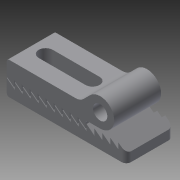
# Autodesk Inventor part: CableClpam
Saved by Autodesk Inventor 2015 (Build 190159000, 159)
## iProperties
Created: 2014-11-13
Part Number: CableClpam
Material: Generic
Document SubType Name: Modeling
Designer: rawrdong
Density: 1 g/cm^3
Appearance: Default
Author: rawrdong
Autodesk Inventor part; units mm, degrees
ref_plane "YZ Plane" through (0, 0, 0) normal (1, 0, 0) x (0, 1, 0)
ref_plane "XZ Plane" through (0, 0, 0) normal (0, 1, 0) x (-1, 0, 0)
ref_plane "XY Plane" through (0, 0, 0) normal (0, 0, 1) x (1, 0, 0)
sketch "Sketch1" plane through (0, 0, 0) normal (0, 1, 0) x (-1, 0, 0)
  line L0 (1.1699, 0) -> (26.6699, 0)
  line L1 (26.6699, 0) -> (26.6699, 2)
  line L2 (26.6699, 2) -> (9.6699, 2)
  line L3 (26.6699, 2) -> (26.6699, 3.3)
  line L4 (26.6699, 3.3) -> (24.9699, 2)
  line L5 (26.6699, 2) -> (24.9699, 2)
  line L6 (24.9699, 2) -> (24.9699, 3.3)
  line L7 (24.9699, 3.3) -> (23.2699, 2)
  line L8 (24.9699, 2) -> (23.2699, 2)
  line L9 (23.2699, 2) -> (23.2699, 3.3)
  line L10 (23.2699, 3.3) -> (21.5699, 2)
  line L11 (23.2699, 2) -> (21.5699, 2)
  line L12 (21.5699, 2) -> (21.5699, 3.3)
  line L13 (21.5699, 3.3) -> (19.8699, 2)
  line L14 (21.5699, 2) -> (19.8699, 2)
  line L15 (19.8699, 2) -> (19.8699, 3.3)
  line L16 (19.8699, 3.3) -> (18.1699, 2)
  line L17 (19.8699, 2) -> (18.1699, 2)
  line L18 (18.1699, 2) -> (18.1699, 3.3)
  line L19 (18.1699, 3.3) -> (16.4699, 2)
  line L20 (18.1699, 2) -> (16.4699, 2)
  line L21 (16.4699, 2) -> (16.4699, 3.3)
  line L22 (16.4699, 3.3) -> (14.7699, 2)
  line L23 (16.4699, 2) -> (14.7699, 2)
  line L24 (14.7699, 2) -> (14.7699, 3.3)
  line L25 (14.7699, 3.3) -> (13.0699, 2)
  line L26 (14.7699, 2) -> (13.0699, 2)
  line L27 (13.0699, 2) -> (13.0699, 3.3)
  line L28 (13.0699, 3.3) -> (11.3699, 2)
  line L29 (13.0699, 2) -> (11.3699, 2)
  line L30 (11.3699, 2) -> (11.3699, 3.3)
  line L31 (11.3699, 3.3) -> (9.6699, 2)
  line L32 (11.3699, 2) -> (9.6699, 2)
  line L33 (9.6699, 2) -> (9.6699, 3.3)
  line L34 (9.6699, 3.3) -> (7.9699, 2)
  line L35 (9.6699, 2) -> (7.9699, 2)
  line L36 (7.9699, 2) -> (7.9699, 3.3)
  line L37 (7.9699, 3.3) -> (6.2699, 2)
  line L38 (7.9699, 2) -> (6.2699, 2)
  line L39 (6.2699, 2) -> (6.2699, 3.3)
  line L40 (6.2699, 3.3) -> (4.5699, 2)
  line L41 (6.2699, 2) -> (4.5699, 2)
  line L42 (4.5699, 2) -> (4.5699, 3.3)
  line L43 (4.5699, 3.3) -> (2.8699, 2)
  line L44 (4.5699, 2) -> (2.8699, 2)
  line L45 (2.8699, 2) -> (2.8699, 3.3)
  line L46 (2.8699, 3.3) -> (1.1699, 2)
  line L47 (2.8699, 2) -> (1.1699, 2)
  line L48 (1.1699, 2) -> (1.1699, 0)
  line L49 (1.1699, 2) -> (26.6699, 2)
  line L50 (26.6699, 2) -> (26.6699, 0)
  line L51 (26.6699, 0) -> (1.1699, 0)
  line L52 (1.1699, 0) -> (1.1699, 2)
  point P0 (0, 0)
  dimension "d7" = 1.3
  dimension "d8" = 2
  dimension "d11" = 1.7
  dimension "d14" = 1.7
  constraints: 106 end point, 3 horizontal, 3 parallel, 3 perpendicular, 1 coincident, 1 collinear, 1 point on line, 1 vertical, 85 other
  measures "d7" distance of L1.end L3.end
  measures "d8" distance of L0.end L1.end
  measures "d11" distance from line of L3 L4.end
  measures "d14" distance of L3.end L7.start
extrude "Extrusion1" add sketch "Sketch1" along normal blind 10
sketch "Sketch2" plane through (0, 10, 0) normal (0, 1, 0) x (1, 0, 0)
  line L0 (-19.8699, -3.3) -> (-18.1699, -2) projected
  line L1 (-18.1699, -2) -> (-18.1699, -3.3) projected
  line L2 (-18.1699, -3.3) -> (-16.4699, -2) projected
  line L3 (-16.4699, -2) -> (-16.4699, -3.3) projected
  line L4 (-16.4699, -3.3) -> (-14.7699, -2) projected
  line L5 (-14.7699, -2) -> (-14.7699, -3.3) projected
  line L6 (-14.7699, -3.3) -> (-13.0699, -2) projected
  line L7 (-13.0699, -2) -> (-13.0699, -3.3) projected
  line L8 (-13.0699, -3.3) -> (-11.3699, -2) projected
  line L9 (-11.3699, -2) -> (-11.3699, -3.3) projected
  line L10 (-11.3699, -3.3) -> (-9.6699, -2) projected
  line L11 (-9.8699, -2.4047) -> (-11.5699, -3.7047)
  line L12 (-11.5699, -3.7047) -> (-11.5699, -2.4047)
  line L13 (-11.5699, -2.4047) -> (-13.2699, -3.7047)
  line L14 (-13.2699, -3.7047) -> (-13.2699, -2.4047)
  line L15 (-13.2699, -2.4047) -> (-14.9699, -3.7047)
  line L16 (-14.9699, -3.7047) -> (-14.9699, -2.4047)
  line L17 (-14.9699, -2.4047) -> (-16.6699, -3.7047)
  line L18 (-16.6699, -3.7047) -> (-16.6699, -2.4047)
  line L19 (-16.6699, -2.4047) -> (-18.3699, -3.7047)
  line L20 (-18.3699, -3.7047) -> (-18.3699, -2.4047)
  line L21 (-18.3699, -2.4047) -> (-20.0699, -3.7047)
  line L22 (-10.9918, -6.9047) -> (-26.6699, -6.9047)
  line L23 (-21.5699, -3.3) -> (-19.8699, -2) projected
  line L24 (-19.8699, -2) -> (-19.8699, -3.3) projected
  line L25 (-20.0699, -2.4047) -> (-20.0699, -3.7047)
  line L26 (-20.0699, -2.4047) -> (-21.7699, -3.7047)
  circle A0 centre (-6.7492, -6.9047) radius 1.525
  circle A1 centre (-6.7492, -6.9047) radius 3
  line L27 (-8.8705, -9.026) -> (-10.9918, -6.9047)
  line L28 (-6.7492, -3.9047) -> (-9.8699, -3.9047)
  line L29 (-9.8699, -2.4047) -> (-9.8699, -3.9047)
  line L30 (-9.6699, -2) -> (-9.6699, -3.3) projected
  line L31 (-26.6699, -3.3) -> (-24.9699, -2) projected
  line L32 (-24.9699, -2) -> (-24.9699, -3.3) projected
  line L33 (-24.9699, -3.3) -> (-23.2699, -2) projected
  line L34 (-23.2699, -2) -> (-23.2699, -3.3) projected
  line L35 (-23.2699, -3.3) -> (-21.5699, -2) projected
  line L36 (-4.5699, -2) -> (-4.5699, -3.3) projected
  line L37 (-21.7699, -2.4047) -> (-23.4699, -3.7047)
  line L38 (-23.4699, -3.7047) -> (-23.4699, -2.4047)
  line L39 (-23.4699, -2.4047) -> (-25.1699, -3.7047)
  line L40 (-25.1699, -3.7047) -> (-25.1699, -2.4047)
  line L41 (-25.1699, -2.4047) -> (-26.6699, -3.5518)
  line L42 (-21.7699, -2.4047) -> (-21.7699, -3.7047)
  line L43 (-6.2699, -2) -> (-6.2699, -3.3) projected
  line L44 (-26.6699, -3.5518) -> (-26.6699, -6.9047)
  dimension "d22" = 0.2
  dimension "d23" = 0.2
  dimension "d53" = 3.05
  dimension "d54" = 6
  dimension "d55" = 0.2
  dimension "d71" = 0.2
  dimension "d76" = 135
  constraints: 48 end point, 7 parallel, 5 horizontal alignment, 2 centre point, 2 horizontal, 2 point on circle, 2 tangent, 1 coincident, 12 other
  measures "d22" distance between parallel lines of L4 L17
  measures "d23" distance between parallel lines of L10 L11
  measures "d53" diameter of A0
  measures "d54" diameter of A1
  measures "d55" distance from line of L11.end L28
  measures "d71" distance between parallel lines of L30 L29
  measures "d76" angle of L22 L27
extrude "Extrusion2" add sketch "Sketch2" against normal blind 10
sketch "Sketch13" plane through (-1.1699, 0, 0) normal (0, 0, -1) x (-1, 0, 0)
  line L0 (25.5, 0) -> (25.5, 10) projected
  line L1 (0, 10) -> (25.5, 10) projected
  circle A0 centre (12.75, 5) radius 1.5
  point P0 (-1.1699, 0)
  point P1 (12.75, 10)
  point P2 (25.5, 5)
  dimension "d73" = 3
  constraints: 2 midpoint, 1 centre point, 1 horizontal alignment, 1 vertical alignment
  measures "d73" diameter of A0
extrude "Extrusion13" cut sketch "Sketch13" against normal up to next
sketch "Sketch4" plane through (-10.302, 0, 6.9047) normal (0, 0, 1) x (1, 0, 0)
  line L0 (-16.3678, 10) -> (-0.6898, 10) projected
  line L1 (-13.0678, 5) -> (-3.0678, 5) construction
  line L2 (-13.0678, 3.5) -> (-3.0678, 3.5)
  line L3 (-3.0678, 6.5) -> (-13.0678, 6.5)
  arc A0 (-13.0678, 6.5) -> (-13.0678, 3.5) centre (-13.0678, 5) ccw
  arc A1 (-3.0678, 3.5) -> (-3.0678, 6.5) centre (-3.0678, 5) ccw
  line L4 (-16.3678, 10) -> (-16.3678, 0) projected
  circle A2 centre (-3.6178, 5) radius 1.5 projected
  point P0 (-8.0678, 5)
  point P1 (-8.0678, 10)
  point P2 (-16.3678, 5)
  dimension "d32" = 3
  dimension "d35" = 10
  constraints: 8 end point, 4 point on circle, 4 tangent, 2 centre point, 2 midpoint, 2 parallel, 1 horizontal alignment, 1 vertical alignment
  measures "d32" distance between parallel lines of L2 L3
  measures "d35" distance of L1.start L1.end
extrude "Extrusion4" cut sketch "Sketch4" against normal up to next
fillet "Fillet5" radius 2.5 1 edges at (-10.9918, 5, 6.9047)
fillet "Fillet6" radius 0.5 3 edges at (-26.6699, 5, 6.9047) (-26.6699, 5, 0) (-9.8699, 5, 3.9047)
fillet "Fillet9" radius 1 2 edges at (-1.1699, 10, 1) (-1.1699, 0, 1)
sketch "Sketch11" plane through (-23.3699, 5.4, 6.5462) normal (0, -1, 0) x (1, 0, 0)
  line L0 (8.4, -2.8415) -> (10, -4.065) projected
  line L1 (8.4, -4.1415) -> (8.4, -2.8415) projected
  line L2 (6.7, -2.8415) -> (8.4, -4.1415) projected
  line L3 (6.7, -4.1415) -> (6.7, -2.8415) projected
  line L4 (5, -2.8415) -> (6.7, -4.1415) projected
  line L5 (5, -4.1415) -> (5, -2.8415) projected
  line L6 (3.3, -2.8415) -> (5, -4.1415) projected
  line L7 (0, 0) -> (0, -2.9179) projected
  line L8 (10, 0) -> (0, 0) projected
  line L9 (10, 0) -> (10, -4.065) projected
  line L10 (3.3, -4.1415) -> (3.3, -2.8415) projected
  line L11 (1.6, -2.8415) -> (3.3, -4.1415) projected
  line L12 (1.6, -4.1415) -> (1.6, -2.8415) projected
  line L13 (0, -2.9179) -> (1.6, -4.1415) projected
  point P0 (23.3699, -6.5462)
sketch "Sketch12" plane through (-8.6125, 4.4, 3.9015) normal (0, -1, 0) x (0.9999994, 0, -0.0010725)
  circle A0 centre (2.2691, 2.5) radius 1.5 projected
  arc A1 (2.2691, 0) -> (0.4995, 4.2659) centre (2.2691, 2.5) ccw projected
  line L0 (0, 3.7653) -> (0.4995, 4.2659) projected
  line L1 (0, 0) -> (0, 3.7653) projected
  line L2 (2.2691, 0) -> (0, 0) projected
  line L3 (0.2497, 4.0156) -> (0.2497, 0)
  point P0 (8.6166, -3.8923)
  constraints: 2 end point, 1 midpoint, 1 perpendicular, 1 point on line
body "Solid1"
